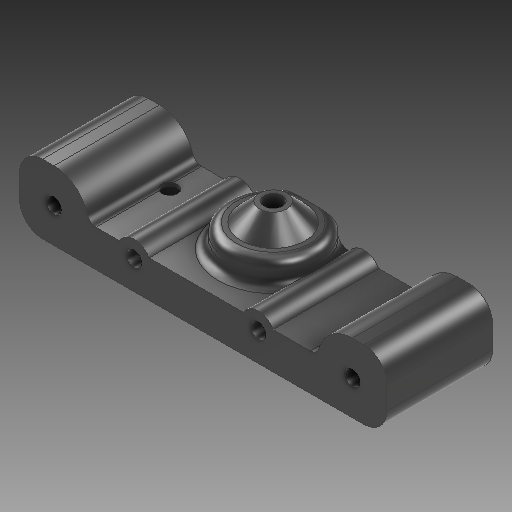
# Autodesk Inventor part: Lower Extruder Block
Saved by Autodesk Inventor 2020.2 (Build 242310000, 310)
## iProperties
Created: 2020-03-20
Part Number: Lower Extruder Block
Material: ABS Plastic
Document SubType Name: Modeling
Designer: rah75
Density: 1.06 g/cm^3
Appearance: Satin - Black
Author: rah75
Title: Lower Extruder Block
Autodesk Inventor part; units mm, degrees
ref_plane "YZ Plane" through (0, 0, 0) normal (1, 0, 0) x (0, 1, 0)
ref_plane "XZ Plane" through (0, 0, 0) normal (0, 1, 0) x (-1, 0, 0)
ref_plane "XY Plane" through (0, 0, 0) normal (0, 0, 1) x (1, 0, 0)
sketch "Sketch1" plane through (0, 0, 0) normal (0, 0, 1) x (1, 0, 0)
  line L0 (-32.5, 0) -> (32.5, 0) construction
  line L1 (-32.5, -7.5) -> (32.5, -7.5)
  line L2 (32.5, 7.5) -> (-32.5, 7.5)
  arc A0 (-32.5, 7.5) -> (-32.5, -7.5) centre (-32.5, 0) ccw
  arc A1 (32.5, -7.5) -> (32.5, 7.5) centre (32.5, 0) ccw
  arc A2 (-25.0167, 0.5) -> (-32.5, 7.5) centre (-32.5, 0) ccw
  arc A3 (32.5, 7.5) -> (25.0167, 0.5) centre (32.5, 0) ccw
  line L3 (-25.0167, 0.5) -> (25.0167, 0.5)
  point P0 (0, 0)
  point P1 (-32.5, 7.5)
  dimension "d0" = 15
  dimension "d1" = 65
  dimension "d3" = 8
  constraints: 10 end point, 8 point on circle, 6 tangent, 4 centre point, 2 concentric, 2 parallel, 1 horizontal, 1 midpoint, 1 point on line
  measures "d0" diameter of A1
  measures "d1" distance of L0.start L0.end
  measures "d3" distance between parallel lines of L1 L3
extrude "Extrusion1" add sketch "Sketch1" along normal mid plane 23 contours A0 A2 L3 A3 A1 L1
sketch "Sketch2" plane through (-32.5, 0.5, 11.5) normal (0, -1, 0) x (1, 0, 0)
  line L0 (65, -23) -> (0, -23) projected
  circle A0 centre (32.5, -15.25) radius 10
  point P0 (32.5, -11.5)
  point P1 (38.8196, -23)
  point P2 (26.1804, -23)
  dimension "d6" = 7.75
  dimension "d14" = 20
  constraints: 1 centre point, 1 coincident, 1 vertical alignment
  measures "d6" distance from line of L0 point (32.5, -15.25)
  measures "d14" diameter of A0
extrude "Extrusion2" add sketch "Sketch2" against normal blind 5 contours L0 A0 picked at (30.3633, -19.1493)
sketch "Sketch3" plane through (-32.5, -7.5, 11.5) normal (0, -1, 0) x (1, 0, 0)
  arc A0 (38.8196, -23) -> (26.1804, -23) centre (32.5, -15.25) ccw projected
  point P0 (32.5, -11.5)
  constraints: 1 coincident
hole "Hole2" at (0, -7.5, -3.75) direction (0, 1, 0) diameter 4 end through all start extended yes counterbore diameter 17 counterbore depth 10
sketch "Sketch4" plane through (-32.5, 5.5, 11.5) normal (0, 1, 0) x (1, 0, 0)
  circle A0 centre (32.5, 15.25) radius 2 projected
  circle A1 centre (32.5, 15.25) radius 5
  point P0 (32.5, 11.5)
  dimension "d24" = 10
  constraints: 1 centre point, 1 coincident
  measures "d24" diameter of A1
extrude "Extrusion3" add sketch "Sketch4" along normal blind 4
fillet "Fillet1" radius 2 4 edges at (0, 0.5, 6.25) (0, 5.5, 6.25) (25.0167, 0.5, 0) (-25.0167, 0.5, 0)
sketch "Sketch5" plane through (-32.5, -7.5, 11.5) normal (0, -1, 0) x (1, 0, 0)
  circle A0 centre (32.5, -15.25) radius 2 projected
  line L0 (63, -2.75) -> (2, -2.75)
  line L1 (2, -2.75) -> (2, -27.75)
  line L2 (2, -27.75) -> (63, -27.75)
  line L3 (63, -27.75) -> (63, -2.75)
  line L4 (63, -2.75) -> (2, -27.75) construction
  line L5 (2, -2.75) -> (63, -27.75) construction
  point P0 (32.5, -11.5)
  dimension "d28" = 61
  dimension "d29" = 12.5
  constraints: 12 end point, 2 midpoint, 2 parallel, 1 horizontal, 1 perpendicular
  measures "d28" distance of L2.end L1.end
  measures "d29" distance from line of A0.centre L0
extrude "Extrusion4" cut sketch "Sketch5" against normal blind 2.5
sketch "Sketch6" plane through (0, 0, -11.5) normal (0, 0, -1) x (-1, 0, 0)
  arc A0 (-25.2644, 1.9737) -> (-32.5, -7.5) centre (-32.5, 0) ccw projected
  arc A1 (32.5, -7.5) -> (25.2644, 1.9737) centre (32.5, 0) ccw projected
  point P0 (0, 0)
  point P1 (-32.5, 0)
  constraints: 2 coincident
hole "Hole3" at (32.5, 0, -11.5) at (-32.5, 0, -11.5) direction (0, 0, 1) diameter 3.4 end through all start extended yes clearance for "Socket Head Cap Screw" size "M3" standard "Ansi Metric M Profile"
sketch "Sketch7" plane through (0, 0, 11.5) normal (0, 0, 1) x (1, 0, 0)
  circle A0 centre (32.5, 0) radius 1.7 projected
  circle A1 centre (-32.5, 0) radius 1.7 projected
  arc A2 (32.5, -7.5) -> (25.2644, 1.9737) centre (32.5, 0) ccw projected
  arc A3 (23.3348, 0.5) -> (25.2644, 1.9737) centre (23.3348, 2.5) ccw projected
  line L0 (23.3348, 0.5) -> (-23.3348, 0.5) projected
  arc A4 (-25.2644, 1.9737) -> (-23.3348, 0.5) centre (-23.3348, 2.5) ccw projected
  arc A5 (-25.2644, 1.9737) -> (-32.5, -7.5) centre (-32.5, 0) ccw projected
  line L1 (-32.5, -7.5) -> (32.5, -7.5) projected
  arc A6 (-25.2644, 1.9737) -> (-32.5, -7.5) centre (-32.5, 0) ccw projected
  line L2 (-32.5, 7.5) -> (-35, 7.5)
  line L3 (-40, 2.5) -> (-40, -2.5)
  line L4 (-35, -7.5) -> (-32.5, -7.5)
  arc A7 (-35, 7.5) -> (-40, 2.5) centre (-35, 2.5) ccw
  arc A8 (-40, -2.5) -> (-35, -7.5) centre (-35, -2.5) ccw
  point P0 (0, 0)
  point P1 (-40, 0)
  dimension "d39" = 5
  constraints: 7 tangent, 6 end point, 5 point on circle, 2 centre point, 1 equal radius, 1 horizontal, 1 parallel, 1 vertical
  measures "d39" radius of A7
extrude "Extrusion5" add sketch "Sketch7" against normal up to surface (23 mm away) contours L4 A8 L3 A5 | L3 A7 L2 A5
mirror "Mirror1" about plane through (0, 0, 0) normal (1, 0, 0) of "Extrusion5"
sketch "Sketch8" plane through (-32.5, -5, 11.5) normal (0, -1, 0) x (1, 0, 0)
  circle A0 centre (32.5, -15.25) radius 2 projected
  circle A1 centre (58, -15.25) radius 2.65
  circle A2 centre (10, -15.25) radius 2.65
  point P0 (32.5, -11.5)
  dimension "d42" = 25.5
  dimension "d43" = 22.5
  dimension "d44" = 5.3
  dimension "d45" = 5.3
  constraints: 2 centre point, 2 coincident, 2 horizontal alignment
  measures "d42" distance of point (58, -15.25) A0.centre
  measures "d43" distance of point (10, -15.25) A0.centre
  measures "d44" diameter of A1
  measures "d45" diameter of A2
hole "Hole4" at (25.5, -5, -3.75) at (-22.5, -5, -3.75) direction (0, 1, 0) diameter 5 depth 4.75 start extended yes countersink diameter 5.4 countersink angle 8
sketch "Sketch9" plane through (25.5, -0.25, -3.75) normal (0, -1, 0) x (1, 0, 0)
  circle A0 centre (0, 0) radius 2.7 projected
  circle A1 centre (-48, 0) radius 2.5 projected
  point P0 (-25.5, 3.75)
  constraints: 2 coincident
hole "Hole5" at (25.5, -0.25, -3.75) at (-22.5, -0.25, -3.75) direction (0, 1, 0) diameter 3.4 depth 9.5 start extended yes clearance for "Socket Head Cap Screw" size "M3" standard "Ansi Metric M Profile"
sketch "Sketch11" plane through (0, 0, -11.5) normal (0, 0, -1) x (-1, 0, 0)
  circle A0 centre (-12, -1.3) radius 2.7
  circle A1 centre (15, -1.3) radius 2.7
  line L0 (-30.5, -5) -> (-3.4911, -5) projected
  circle A2 centre (-12, -1.3) radius 3.7
  circle A3 centre (15, -1.3) radius 3.7
  line L1 (30.5, -7.5) -> (-30.5, -7.5) projected
  point P0 (0, 0)
  dimension "d71" = 5.4
  dimension "d72" = 5.4
  dimension "d73" = 15
  dimension "d74" = 12
  dimension "d76" = 1
  dimension "d94" = 6.2
  constraints: 4 centre point, 1 equal radius, 1 horizontal alignment
  measures "d71" diameter of A0
  measures "d72" diameter of A1
  measures "d73" horizontal distance of A1.centre point (0, 0)
  measures "d74" horizontal distance of A0.centre point (0, 0)
  measures "d76" radial gap between concentric circles of A0 A2
  measures "d94" distance from line of A0.centre L1
extrude "Extrusion6" add sketch "Sketch11" against normal up to surface (23 mm away) contours A0 | A1 | A2 | A3
sketch "Sketch12" plane through (0, 0, -11.5) normal (0, 0, -1) x (-1, 0, 0)
  arc A0 (-8.7792, 0.5211) -> (-15.2326, 0.5) centre (-12, -1.3) ccw projected
  arc A1 (18.2326, 0.5) -> (11.7674, 0.5) centre (15, -1.3) ccw projected
  point P0 (0, 0)
  point P1 (-13.7674, 0.5)
  constraints: 2 coincident
hole "Hole7" at (12, -1.3, -11.5) at (-15, -1.3, -11.5) direction (0, 0, 1) diameter 3.4 end through all start extended yes clearance for "Socket Head Cap Screw" size "M3" standard "Ansi Metric M Profile"
fillet "Fillet2" radius 0.75 2 edges at (3.4911, -1.25, -11.5) (-3.4911, -1.25, -11.5)
chamfer "Chamfer1" distance 2 angle 45 2 edges at (-5, 5.5, -3.75) (-5, 9.5, -3.75)
sketch "Sketch15" plane through (0, 2.5, -3.75) normal (0, -1, 0) x (1, 0, 0)
  circle A0 centre (0, 0) radius 2 projected
  circle A1 centre (0, 0) radius 1.25
  point P0 (0, 3.75)
  dimension "d103" = 0.75
  constraints: 1 centre point
  measures "d103" radial gap between concentric circles of A0 A1
extrude "Extrusion7" add sketch "Sketch15" against normal blind 0.75
sketch "Sketch16" plane through (0, 2.5, -3.75) normal (0, -1, 0) x (1, 0, 0)
  circle A0 centre (0, 0) radius 1.25 projected
  line L0 (6.0467, -7.75) -> (-6.0467, -7.75) projected
  arc A1 (5.5564, -6.4324) -> (6.0467, -7.75) centre (6.0467, -7) ccw projected
  arc A2 (5.5564, -6.4324) -> (-5.5564, -6.4324) centre (0, 0) ccw projected
  arc A3 (-6.0467, -7.75) -> (-5.5564, -6.4324) centre (-6.0467, -7) ccw projected
  point P0 (0, 3.75)
extrude "Extrusion8" cut sketch "Sketch16" along normal blind 10
body "Solid1"
